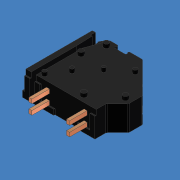
# Autodesk Inventor part: Wago 745-851 (76A) Black
Saved by Autodesk Inventor 2012 (Build 160160000, 160)
## iProperties
Category: PARTsolutions
Company: Team 801
Created: 2007-09-01
Part Number: Wago 745-851 (76A) Black
Catalog Web Link: www.team801.org
Description: 745-851/006-000 - MODULAR PCB TERMINAL BLOCK 4 SOLDER PINS/POLE PIN SPACING 10 MM / 0.394 IN
Document SubType Name: Modeling
Designer: Jeffrey M
Mass: 6.81841 g
Surface Area: 34.4261 cm^2
Volume: 6.81841 cm^3
Density: 1 g/cm^3
Material: Default
NB: 745-851/006-000
NN: 745-851/006-000
NT: MODULAR PCB TERMINAL BLOCK 4 SOLDER PINS/POLE PIN SPACING 10 MM / 0.394 IN
NBSYN: $BESTNR.
LINA: 745-851/006-000
BESTNR: 745-851/006-000
QUERSCHNITT1: 0.2 - 16
QUERSCHNITT2: 24 - 06
ABISOLIERLAENGE: 12 - 13
SPANNUNG: 250
BEMESSSTOSSSPG: 4
VERSCHMUTZGRAD: 3
STROM: 57
RM: 10.00
P: 1
HOEHE: 27.00
BREITE: 10.00
TIEFE: 33.40
ANZAHLKLEMMSTEL: 1
ANZAHLPOTENTIAL: 1
FARBE: grau
GEWICHT: 8.938
EAN: 4044918303149
BOHRLOCHDURCHM: 2,2 + 0,1 mm
RGB: 0.67,0.67,0.67,0
KT: DUMMY
PSOL_IDENT_0: {\\partserver001.servicenet\dplatte\cadenas\23d-libs\wago\pg04\serie745\0745-0851_0006_0999-0962.prj
PSOL_IDENT_1: },173 {VTYP=3D},{NB=745-851/006-000},{LINA=745-851/006-000},{NN=745-851/006-000},{DATE=10.04.2007 09
PSOL_IDENT_2: :25:18},{GEOMDATE=13.06.2006},{VERSION=},{LINEID=160},{LINESUBID=-1},{WBVAR=}  {NB=745-851/006-000},
PSOL_IDENT_3: {LINA=745-851/006-000},{KT=DUMMY},{BESTNR=745-851/006-000},{QUERSCHNITT1=0.2 - 16},{QUERSCHNITT2=24
PSOL_IDENT_4: - 06},{ABISOLIERLAENGE=12 - 13},{SPANNUNG=250},{BEMESSSTOSSSPG=4},{VERSCHMUTZGRAD=3},{STROM=57},{RM=
PSOL_IDENT_5: 10.00},{P=1},{HOEHE=27.00},{BREITE=10.00},{TIEFE=33.40},{ANZAHLKLEMMSTEL=1},{ANZAHLPOTENTIAL=1},{FAR
PSOL_IDENT_6: BE=grau},{GEWICHT=8.938},{EAN=4044918303149},{BOHRLOCHDURCHM=2,2 + 0,1 mm},{RGB=0.67,0.67,0.67,0}
Title: Wago 745-851 (76A)
Author: Jeffrey M
Comments: MODULAR PCB TERMINAL BLOCK 4 SOLDER PINS/POLE PIN SPACING 10 MM / 0.394 IN
Autodesk Inventor part; units mm, degrees
ref_plane "YZ Plane" through (0, 0, 0) normal (1, 0, 0) x (0, 1, 0)
ref_plane "XZ Plane" through (0, 0, 0) normal (0, 1, 0) x (-1, 0, 0)
ref_plane "XY Plane" through (0, 0, 0) normal (0, 0, 1) x (1, 0, 0)
sketch "Skizze_1" plane through (0, 0, 0) normal (0, 0, 1) x (1, 0, 0)
  line L0 (-23.8, 0) -> (4.2, 0)
  line L1 (4.2, 0) -> (4.2, 4.0858)
  arc A0 (4.4929, 4.7929) -> (4.2, 4.0858) centre (5.2, 4.0858) ccw
  line L2 (4.4929, 4.7929) -> (8.4071, 8.7071)
  arc A1 (8.4071, 8.7071) -> (8.7, 9.4142) centre (7.7, 9.4142) ccw
  line L3 (8.7, 9.4142) -> (8.7, 14.0815)
  arc A2 (8.7, 14.0815) -> (8.4071, 14.7886) centre (7.7, 14.0815) ccw
  line L4 (8.4071, 14.7886) -> (-3.5114, 26.7071)
  arc A3 (-3.5114, 26.7071) -> (-4.2185, 27) centre (-4.2185, 26) ccw
  line L5 (-4.2185, 27) -> (-16.4499, 27)
  arc A4 (-16.4499, 27) -> (-16.9197, 26.671) centre (-16.4499, 26.5) ccw
  line L6 (-16.9197, 26.671) -> (-19.5556, 19.429)
  arc A5 (-20.0255, 19.1) -> (-19.5556, 19.429) centre (-20.0255, 19.6) ccw
  line L7 (-20.0255, 19.1) -> (-21.2413, 19.1)
  arc A6 (-21.741, 19.5826) -> (-21.2413, 19.1) centre (-21.2413, 19.6) ccw
  line L8 (-21.741, 19.5826) -> (-21.9899, 26.7105)
  arc A7 (-21.9899, 26.7105) -> (-22.2897, 27) centre (-22.2897, 26.7) ccw
  line L9 (-22.2897, 27) -> (-23.5, 27)
  arc A8 (-23.5, 27) -> (-23.8, 26.7) centre (-23.5, 26.7) ccw
  line L10 (-23.8, 26.7) -> (-23.8, 0)
  constraints: 22 end point, 18 point on circle, 9 centre point
extrude "Extrusion1" add sketch "Skizze_1" along normal blind 10
sketch "Skizze_2" plane through (0, 0, 0) normal (0, 0, 1) x (1, 0, 0)
  arc A0 (-13.5012, 26.3457) -> (-13.81, 27) centre (-13.81, 26.6) ccw
  line L0 (-13.5012, 26.3457) -> (-13.6282, 26.1915)
  arc A1 (-13.6282, 26.1915) -> (-13.3475, 25.3998) centre (-13.25, 25.88) ccw
  line L1 (-13.3475, 25.3998) -> (-13.25, 25.38)
  line L2 (-13.25, 25.38) -> (-9.35, 25.38)
  line L3 (-9.35, 25.38) -> (-9.2525, 25.3998)
  arc A2 (-9.2525, 25.3998) -> (-8.9718, 26.1915) centre (-9.35, 25.88) ccw
  line L4 (-8.9718, 26.1915) -> (-9.0988, 26.3457)
  arc A3 (-8.79, 27) -> (-9.0988, 26.3457) centre (-8.79, 26.6) ccw
  line L5 (-8.79, 27) -> (-13.81, 27)
  constraints: 12 end point, 8 point on circle, 4 centre point
extrude "Extrusion2" cut sketch "Skizze_2" along normal blind 10
sketch "Skizze_4" plane through (0, 0, 0) normal (0, 0, 1) x (1, 0, 0)
  line L0 (-24.7, 0) -> (-22.4, 0)
  line L1 (-22.4, 0) -> (-22.4, 27)
  line L2 (-22.4, 27) -> (-23.5, 27)
  arc A0 (-23.5, 27) -> (-24.7, 25.8) centre (-23.5, 25.8) ccw
  line L3 (-24.7, 25.8) -> (-24.7, 17.9727)
  line L4 (-24.7, 17.9727) -> (-23.8, 15.5)
  line L5 (-23.8, 15.5) -> (-23.8, 8)
  line L6 (-23.8, 8) -> (-24.7, 5.5273)
  line L7 (-24.7, 5.5273) -> (-24.7, 0)
  constraints: 16 end point, 2 point on circle, 1 centre point
extrude "Extrusion3" add sketch "Skizze_4" along normal blind 2.4
sketch "Skizze_3" plane through (0, 0, 10) normal (0, 0, 1) x (1, 0, 0)
  line L0 (-22, 27) -> (-21.7, 18.4091)
  line L1 (-21.7, 18.4091) -> (-21.7, 0)
  line L2 (-21.7, 0) -> (-19.7, 0)
  line L3 (-19.7, 0) -> (-19.7, 27)
  line L4 (-19.7, 27) -> (-22, 27)
  constraints: 10 end point
extrude "Extrusion4" cut sketch "Skizze_3" against normal blind 8.8
sketch "Skizze_5" plane through (0, 0, 10) normal (0, 0, 1) x (1, 0, 0)
  line L0 (-22.6, 27) -> (-22.6, 25.1)
  line L1 (-22.6, 25.1) -> (-21.6, 25.1)
  line L2 (-21.6, 25.1) -> (-21.6, 27)
  line L3 (-21.6, 27) -> (-22.6, 27)
  constraints: 8 end point
extrude "Extrusion5" cut sketch "Skizze_5" against normal blind 7.6
sketch "Skizze_8" plane through (0, 0, 10) normal (0, 0, 1) x (1, 0, 0)
  circle A0 centre (6.4, 10) radius 1
  constraints: 1 centre point
extrude "Extrusion6" add sketch "Skizze_8" along normal blind 1.5
sketch "Skizze_9" plane through (0, 0, 10) normal (0, 0, 1) x (1, 0, 0)
  circle A0 centre (-3, 2.8) radius 1
  constraints: 1 centre point
extrude "Extrusion7" add sketch "Skizze_9" along normal blind 1.5
sketch "Skizze_10" plane through (0, 0, 10) normal (0, 0, 1) x (1, 0, 0)
  circle A0 centre (-18, 2.1) radius 0.8
  constraints: 1 centre point
extrude "Extrusion8" add sketch "Skizze_10" along normal blind 1.5
sketch "Skizze_11" plane through (0, 0, 10) normal (0, 0, 1) x (1, 0, 0)
  circle A0 centre (-17.7, 16.4) radius 1
  constraints: 1 centre point
extrude "Extrusion9" add sketch "Skizze_11" along normal blind 1.5
sketch "Skizze_12" plane through (0, 0, 10) normal (0, 0, 1) x (1, 0, 0)
  circle A0 centre (-15.5, 24.3) radius 1
  constraints: 1 centre point
extrude "Extrusion10" add sketch "Skizze_12" along normal blind 1.5
sketch "Skizze_13" plane through (0, 0, 10) normal (0, 0, 1) x (1, 0, 0)
  circle A0 centre (-13.6, 8.7) radius 0.8
  constraints: 1 centre point
extrude "Extrusion11" add sketch "Skizze_13" along normal blind 1.5
sketch "Skizze_14" plane through (0, 0, 10) normal (0, 0, 1) x (1, 0, 0)
  circle A0 centre (-7.6, 15.3) radius 0.7
  constraints: 1 centre point
extrude "Extrusion12" add sketch "Skizze_14" along normal blind 1.5
sketch "Skizze_15" plane through (0, 0, 10) normal (0, 0, 1) x (1, 0, 0)
  circle A0 centre (-0.6, 20.9) radius 0.8
  constraints: 1 centre point
extrude "Extrusion13" add sketch "Skizze_15" along normal blind 1.5
sketch "Skizze_6" plane through (0, 0, 8.8) normal (0, 0, 1) x (1, 0, 0)
  arc A0 (-19.9598, 25.55) -> (-19.7, 25.1) centre (-19.7, 25.4) ccw
  line L0 (-19.7, 25.1) -> (-19.7, 19.1)
  line L1 (-19.7, 19.1) -> (-15.8, 19.1)
  line L2 (-15.8, 19.1) -> (-15.8, 27)
  line L3 (-15.8, 27) -> (-18.9494, 27)
  arc A1 (-18.9494, 27) -> (-19.2093, 26.85) centre (-18.9494, 26.7) ccw
  line L4 (-19.2093, 26.85) -> (-19.9598, 25.55)
  constraints: 10 end point, 4 point on circle, 2 centre point
extrude "Extrusion14" add sketch "Skizze_6" against normal blind 6.3
sketch "Skizze_7" plane through (0, 0, 0) normal (0, 1, 0) x (-1, 0, 0)
  line L0 (23.8, 7.9) -> (23.8, 10)
  line L1 (23.8, 10) -> (-4.2, 10)
  line L2 (-4.2, 10) -> (-4.2, 7.9)
  line L3 (-4.2, 7.9) -> (-2.2, 7.9)
  line L4 (-2.2, 7.9) -> (-2.2, 2.1)
  line L5 (-2.2, 2.1) -> (2.8, 2.1)
  line L6 (2.8, 2.1) -> (2.8, 0)
  line L7 (2.8, 0) -> (12.2, 0)
  line L8 (12.2, 0) -> (12.2, 2.1)
  line L9 (12.2, 2.1) -> (17.7, 2.1)
  line L10 (17.7, 2.1) -> (17.7, 7.9)
  line L11 (17.7, 7.9) -> (19.7, 7.9)
  line L12 (19.7, 7.9) -> (19.7, 3.5)
  line L13 (19.7, 3.5) -> (21.7, 3.5)
  line L14 (21.7, 3.5) -> (21.7, 7.9)
  line L15 (21.7, 7.9) -> (23.8, 7.9)
  constraints: 32 end point
extrude "Extrusion15" cut sketch "Skizze_7" along normal blind 0.5
sketch "Skizze_16" plane through (0, 0, 5) normal (0, 0, 1) x (1, 0, 0)
  line L0 (3.46, 16.2002) -> (5.2277, 17.9679)
  line L1 (5.2277, 17.9679) -> (8.834, 14.3617)
  line L2 (8.834, 14.3617) -> (7.7026, 14.3617)
  line L3 (7.7026, 14.3617) -> (6.5005, 13.1596)
  line L4 (6.5005, 13.1596) -> (3.46, 16.2002)
  line L5 (3.46, 16.2002) -> (5.2277, 17.9679)
  constraints: 12 end point
revolve "Revolution1" cut sketch "Skizze_16" angle 360 about axis through (3.46, 16.2002, 5) along (-0.7071068, -0.7071068, 0)
sketch "Skizze_17" plane through (0, 0, 5) normal (0, 0, 1) x (1, 0, 0)
  line L0 (-7.0492, 24.5) -> (-4.8398, 24.5)
  line L1 (-4.8398, 24.5) -> (-2.1262, 21.7863)
  line L2 (-2.1262, 21.7863) -> (-0.3584, 23.5541)
  line L3 (-0.3584, 23.5541) -> (-3.8043, 27)
  line L4 (-3.8043, 27) -> (-5.7563, 27)
  arc A0 (-5.4028, 26.1464) -> (-5.7563, 27) centre (-5.7563, 26.5) ccw
  line L5 (-5.4028, 26.1464) -> (-7.0492, 24.5)
  constraints: 12 end point, 2 point on circle, 1 centre point
extrude "Extrusion16" cut sketch "Skizze_17" along normal mid plane 6.5
sketch "Skizze_18" plane through (0, 0, 6.9) normal (0, 0, 1) x (1, 0, 0)
  line L0 (0.8437, 22.352) -> (-0.9241, 20.5842)
  line L1 (-0.9241, 20.5842) -> (-1.7373, 21.3974)
  line L2 (-1.7373, 21.3974) -> (-0.3982, 22.7365)
  line L3 (-0.3982, 22.7365) -> (-0.217, 23.4127)
  line L4 (-0.217, 23.4127) -> (0.8437, 22.352)
  line L5 (0.8437, 22.352) -> (-0.9241, 20.5842)
  constraints: 12 end point
revolve "Revolution2" cut sketch "Skizze_18" angle 360 about axis through (0.8437, 22.352, 6.9) along (0.7071068, 0.7071068, 0)
sketch "Skizze_19" plane through (0, 0, 0) normal (0, 1, 0) x (-1, 0, 0)
  line L0 (0.6, 3.8) -> (-0.6, 3.8)
  line L1 (-0.6, 3.8) -> (-0.6, 2.2)
  line L2 (-0.6, 2.2) -> (0.6, 2.2)
  line L3 (0.6, 2.2) -> (0.6, 3.8)
  constraints: 8 end point
extrude "Extrusion17" add sketch "Skizze_19" along normal mid plane 13
pattern_linear "Rectangular Pattern1" count 2 spacing 15 along (-1, 0, 0) of "Extrusion17"
sketch "Skizze_21" plane through (0, 0, 0) normal (0, 1, 0) x (-1, 0, 0)
  line L0 (0.6, 7.8) -> (-0.6, 7.8)
  line L1 (-0.6, 7.8) -> (-0.6, 6.2)
  line L2 (-0.6, 6.2) -> (0.6, 6.2)
  line L3 (0.6, 6.2) -> (0.6, 7.8)
  constraints: 8 end point
extrude "Extrusion18" add sketch "Skizze_21" along normal mid plane 13
pattern_linear "Rectangular Pattern2" count 2 spacing 15 along (-1, 0, 0) of "Extrusion18"
sketch "Sketch21" plane through (3.46, 16.2002, 5) normal (0.7071068, 0.7071068, 0) x (-0.7071068, 0.7071068, 0)
  circle A0 centre (0, 0) radius 4.3 projected
body "Solid1"
